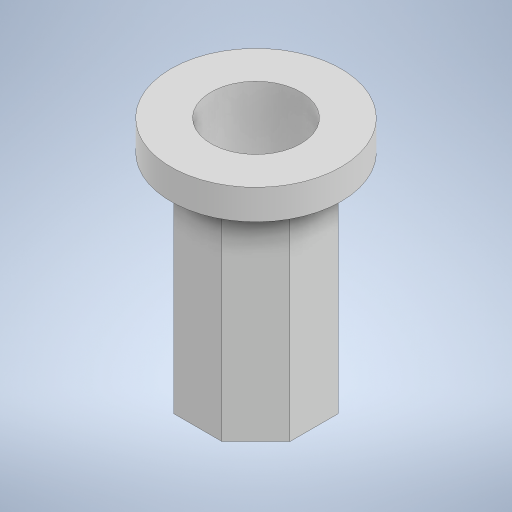
# Autodesk Inventor part: PancakeBearingAdapter
Saved by Autodesk Inventor 2024.3 (Build 283343000, 343)
## iProperties
Created: 2024-12-03
Part Number: PancakeBearingAdapter
Material: Generisch
Document SubType Name: Modeling
Designer: Maximilian Hock
Density: 1 g/cm^3
Appearance: Vorgabe
Author: Maximilian Hock
## iProperties of the stored document MemberDocs/xG1cw44kiPcn4fagy3cfzayvmYe
Created: 2024-12-03
Part Number: PancakeBearingAdapter
Material: Generisch
Document SubType Name: Modeling
Designer: Maximilian Hock
Density: 1 g/cm^3
Appearance: Vorgabe
Author: Maximilian Hock
Autodesk Inventor part; units mm, degrees
ref_plane "YZ Plane" through (0, 0, 0) normal (1, 0, 0) x (0, 1, 0)
ref_plane "XY Plane" through (0, 0, 0) normal (0, 0, 1) x (1, 0, 0)
sketch "Skizze1" plane through (0, 0, 0) normal (0, 0, 1) x (1, 0, 0)
  circle A0 centre (0, 0) radius 7.5 construction
  circle A1 centre (0, 0) radius 3.8803 construction
  circle A2 centre (0, 0) radius 3
  line L0 (0, 3.8803) -> (0, 7.5) construction
  circle A3 centre (0, 0) radius 5.6901
  line L1 (3.8803, -1.6073) -> (1.6073, -3.8803)
  line L2 (1.6073, -3.8803) -> (-1.6073, -3.8803)
  line L3 (-1.6073, -3.8803) -> (-3.8803, -1.6073)
  line L4 (-3.8803, -1.6073) -> (-3.8803, 1.6073)
  line L5 (-3.8803, 1.6073) -> (-1.6073, 3.8803)
  line L6 (-1.6073, 3.8803) -> (1.6073, 3.8803)
  line L7 (1.6073, 3.8803) -> (3.8803, 1.6073)
  line L8 (3.8803, 1.6073) -> (3.8803, -1.6073)
  point P0 (0, 5.6901)
  point P1 (3.8803, 0)
  dimension "d2" = 15
  dimension "d0" = 6
  dimension "d19" = 8.4
  constraints: 18 end point, 7 coincident, 2 centre point, 2 midpoint, 2 point on circle, 2 vertical alignment, 1 horizontal alignment, 1 line through centre, 1 vertical, 21 other
  measures "d0" diameter of A2
  measures "d19" distance of L1.end L5.end
extrude "Extrusion1" add sketch "Skizze1" against normal blind 14 contours L1 L2 L3 L4 L5 L6 L7 L8
extrude "Extrusion2" add sketch "Skizze1" along normal blind 2 contours A3 | L1 L2 L3 L4 L5 L6 L7 L8
ref_plane "Arbeitsebene1" through (0, 17, 0) normal (0, 1, 0) x (-1, 0, 0)
sketch "Skizze4" plane through (0, 17, 0) normal (0, 1, 0) x (-1, 0, 0)
  line L0 (5.6901, 2) -> (-5.6901, 2) construction
  line L1 (5.6901, 0) -> (-5.6901, 0) construction
  line L2 (-5.6901, 2) -> (5.6901, 2) construction
  line L3 (5.6901, 2) -> (5.6901, 0) construction
  line L4 (5.6901, 0) -> (-5.6901, 0) construction
  line L5 (-5.6901, 0) -> (-5.6901, 2) construction
  line L6 (-1.3426, 0.6001) -> (-1.5456, 0.6001)
  line L7 (-1.5456, 0.6001) -> (-1.5456, 0.2464)
  line L8 (-1.5456, 0.2464) -> (-1.909, 0.2464)
  line L9 (-1.909, 0.2464) -> (-1.909, 0.6001)
  line L10 (-1.909, 0.6001) -> (-2.5703, 0.6001)
  line L11 (-2.5703, 0.6001) -> (-2.5703, 0.8797)
  line L12 (-2.5703, 0.8797) -> (-1.9212, 1.75)
  line L13 (-1.9212, 1.75) -> (-1.5456, 1.75)
  line L14 (-1.5456, 1.75) -> (-1.5456, 0.8699)
  line L15 (-1.5456, 0.8699) -> (-1.3426, 0.8699)
  line L16 (-1.3426, 0.8699) -> (-1.3426, 0.6001)
  line L17 (-1.909, 0.8699) -> (-1.909, 1.3805)
  line L18 (-1.909, 1.3805) -> (-2.2895, 0.8699)
  line L19 (-2.2895, 0.8699) -> (-1.909, 0.8699)
  line L20 (-0.8017, 0.25) -> (-1.1578, 0.25)
  line L21 (-1.1578, 0.25) -> (-1.1578, 0.6463)
  line L22 (-1.1578, 0.6463) -> (-0.8017, 0.6463)
  line L23 (-0.8017, 0.6463) -> (-0.8017, 0.25)
  line L24 (0.6157, 0.6001) -> (0.4127, 0.6001)
  line L25 (0.4127, 0.6001) -> (0.4127, 0.2464)
  line L26 (0.4127, 0.2464) -> (0.0492, 0.2464)
  line L27 (0.0492, 0.2464) -> (0.0492, 0.6001)
  line L28 (0.0492, 0.6001) -> (-0.612, 0.6001)
  line L29 (-0.612, 0.6001) -> (-0.612, 0.8797)
  line L30 (-0.612, 0.8797) -> (0.0371, 1.75)
  line L31 (0.0371, 1.75) -> (0.4127, 1.75)
  line L32 (0.4127, 1.75) -> (0.4127, 0.8699)
  line L33 (0.4127, 0.8699) -> (0.6157, 0.8699)
  line L34 (0.6157, 0.8699) -> (0.6157, 0.6001)
  line L35 (0.0492, 0.8699) -> (0.0492, 1.3805)
  line L36 (0.0492, 1.3805) -> (-0.3312, 0.8699)
  line L37 (-0.3312, 0.8699) -> (0.0492, 0.8699)
  line L38 (1.1566, 0.25) -> (0.8004, 0.25)
  line L39 (0.8004, 0.25) -> (0.8004, 0.6463)
  line L40 (0.8004, 0.6463) -> (1.1566, 0.6463)
  line L41 (1.1566, 0.6463) -> (1.1566, 0.25)
  line L42 (2.4889, 0.25) -> (1.4982, 0.25)
  line L43 (1.4982, 0.25) -> (1.4982, 0.5113)
  line L44 (1.4982, 0.5113) -> (1.8142, 0.5113)
  line L45 (1.8142, 0.5113) -> (1.8142, 1.3051)
  line L46 (1.8142, 1.3051) -> (1.4982, 1.3051)
  line L47 (1.4982, 1.3051) -> (1.4982, 1.5494)
  spline S0 degree 2 poles (1.4982, 1.5494) (1.5675, 1.5494) (1.7048, 1.5677) (1.7462, 1.5871) knots 0 0 0 1 2 2 2
  spline S1 degree 2 poles (1.7462, 1.5871) (1.7936, 1.6114) (1.847, 1.6929) (1.8519, 1.7536) knots 0 0 0 1 2 2 2
  line L48 (1.8519, 1.7536) -> (2.1801, 1.7536)
  line L49 (2.1801, 1.7536) -> (2.1801, 0.5113)
  line L50 (2.1801, 0.5113) -> (2.4889, 0.5113)
  line L51 (2.4889, 0.5113) -> (2.4889, 0.25)
  point P0 (0, 0)
  constraints: 2 coincident, 2 other
emboss "Prägen3" sketch "Skizze4" operation cut depth 0.5 direction (0, 1, 0) wrap yes faces at (5.6717, -0.4579, 1.3333)
equation "\"d0\" = AxleDiameter"
equation "\"d3\" = 2 * BearingHeight"
equation "\"AxleDiameter\" = 6"
equation "\"BearingHeight\" = 7"
